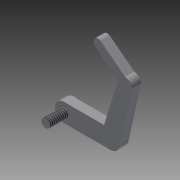
# Autodesk Inventor part: servo_hook
Saved by Autodesk Inventor 2015 SP2 (Build 190223200, 223)
## iProperties
Created: 2016-09-05
Part Number: servo_hook
Material: Generic
Document SubType Name: Modeling
Designer: jm799
Density: 1 g/cm^3
Appearance: Default
Author: jm799
Autodesk Inventor part; units mm, degrees
ref_plane "YZ Plane" through (0, 0, 0) normal (1, 0, 0) x (0, 1, 0)
ref_plane "XZ Plane" through (0, 0, 0) normal (0, 1, 0) x (-1, 0, 0)
ref_plane "XY Plane" through (0, 0, 0) normal (0, 0, 1) x (1, 0, 0)
sketch "Sketch1" plane through (0, 0, 0) normal (0, 1, 0) x (-1, 0, 0)
  circle A0 centre (0, 0) radius 2
  circle A1 centre (0, 0) radius 0.95
  circle A2 centre (-10.0688, 0.0006) radius 1.9997
  line L0 (-0.0618, -1.999) -> (-10.0688, -1.999)
  line L1 (-0.0618, 1.999) -> (-10.0686, 2.0003)
  circle A3 centre (-13.2373, 11.8352) radius 1.5
  line L2 (-8.0691, 0.0006) -> (-11.8022, 12.2717)
  line L3 (-12.0685, 0.0006) -> (-14.7373, 11.8352)
  circle A4 centre (-8.6896, 15.1639) radius 1
  line L4 (-13.2373, 13.3352) -> (-9.2441, 15.9961)
  line L5 (-13.2373, 10.3352) -> (-8.0733, 14.3764)
  dimension "d0" = 4
  dimension "d1" = 1.9
  dimension "d2" = 3
  dimension "d13" = 2
  constraints: 12 end point, 12 point on circle, 5 centre point, 5 tangent, 2 coincident
  measures "d0" diameter of A0
  measures "d1" diameter of A1
  measures "d2" diameter of A3
  measures "d13" diameter of A4
extrude "Extrusion1" add sketch "Sketch1" along normal blind 2 contours A0 | A0 L0 A2 L2 L1 | L2 A2 L1 | L1 A2 L3 A3 L5 L2 | A2 L2 | A2 L2 | L5 A3 L2 | A3 L5 L3 | A3 L5
sketch "Sketch2" plane through (0, 2, 0) normal (0, 1, 0) x (1, 0, 0)
  circle A0 centre (0, 0) radius 0.95
  constraints: 1 centre point, 1 coincident
extrude "Extrusion2" add sketch "Sketch2" against normal blind 6 and the other way blind 0.5
thread "Thread1" size "M2x0.4" class "6g" standard "ANSI Metric M Profile" full length
sketch "Sketch3" plane through (0, 2, 0) normal (0, 1, 0) x (1, 0, 0)
  circle A0 centre (0, 0) radius 1.8246
  constraints: 1 centre point, 1 coincident
extrude "Extrusion3" add sketch "Sketch3" along normal blind 0.3
sketch "Sketch4" plane through (0, 2, 0) normal (0, 1, 0) x (1, 0, 0)
  circle A0 centre (7.388, -16.6186) radius 1
  arc A1 (11.8022, -12.2717) -> (14.7373, -11.8352) centre (13.2373, -11.8352) ccw projected
  line L0 (13.2373, -13.3352) -> (8.002, -17.4079)
  line L1 (8.6774, -2.0002) -> (11.8022, -12.2717) projected
  line L2 (11.6694, -11.8352) -> (6.7559, -15.8438)
  point P0 (0, 0)
  dimension "d14" = 2
  constraints: 4 end point, 3 point on circle, 2 tangent, 1 centre point, 1 point on line
  measures "d14" diameter of A0
extrude "Extrusion4" add sketch "Sketch4" against normal blind 2
body "Solid1"
